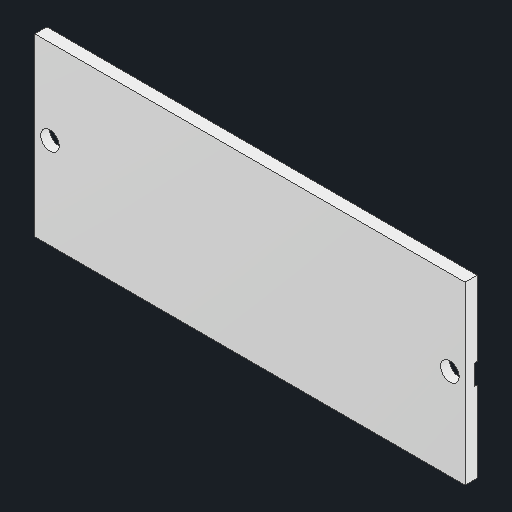
# Autodesk Inventor part: back
Saved by Autodesk Inventor 2023 (Build 270158000, 158)
## iProperties
Created: 2024-05-26
Part Number: back
Material: ABS Plastic
Document SubType Name: Modeling
Designer: szymo
Density: 1.06 g/cm^3
Appearance: Smooth - White
Mass: 4.30907 g
Surface Area: 45.139 cm^2
Volume: 4.06516 cm^3
TOTAL MASS: 0.0
Author: szymo
Autodesk Inventor part; units mm, degrees
ref_plane "YZ Plane" through (0, 0, 0) normal (1, 0, 0) x (0, 1, 0)
ref_plane "XZ Plane" through (0, 0, 0) normal (0, 1, 0) x (-1, 0, 0)
ref_plane "XY Plane" through (0, 0, 0) normal (0, 0, 1) x (1, 0, 0)
sketch "Sketch3" plane through (0, 0, 0) normal (0, 0, 1) x (1, 0, 0)
  line L0 (2.676, 4.0583) -> (2.676, 33.0583) projected
  line L1 (2.676, 4.0583) -> (-2.324, 4.0583) projected
  line L2 (-2.324, 4.0583) -> (-2.324, 33.0583) projected
  line L3 (2.676, 33.0583) -> (-2.324, 33.0583) projected
  line L4 (-68.324, 4.0583) -> (-68.324, 29.5583) projected
  line L5 (-68.324, 33.0583) -> (-63.324, 33.0583) projected
  line L6 (-63.324, 4.0583) -> (-63.324, 33.0583) projected
  line L7 (-68.324, 4.0583) -> (-63.324, 4.0583) projected
  line L8 (2.676, 33.0583) -> (-68.324, 33.0583)
  line L9 (-68.324, 33.0583) -> (-68.324, 4.0583)
  line L10 (-68.324, 4.0583) -> (2.676, 4.0583)
  line L11 (2.676, 4.0583) -> (2.676, 33.0583)
  circle A0 centre (0.176, 19.0583) radius 1.75 projected
  line L12 (-68.324, 29.5583) -> (-68.324, 33.0583) projected
  circle A1 centre (-65.824, 19.0583) radius 1.75 projected
  point P0 (0, 0)
  constraints: 8 end point, 2 parallel, 1 horizontal, 1 perpendicular
extrude "Extrusion2" add sketch "Sketch3" against normal blind 2 contours L1 L2 L3 L0 | L10 L6 L8 L2 | L7 L4 L9 L5 L6 | A0 | A1
sketch "Sketch4" plane through (0, 0, -2) normal (0, 0, -1) x (-1, 0, 0)
  circle A0 centre (-0.176, 19.0583) radius 1.75 projected
  circle A1 centre (65.824, 19.0583) radius 1.75 projected
  point P0 (0, 0)
  constraints: 2 coincident
hole "Hole2" at (0.176, 19.0583, -2) at (-65.824, 19.0583, -2) direction (0, 0, 1) diameter 3.1 end through all counterbore diameter 6 counterbore depth 0.5 clearance for "Countersunk Flat Head Screw ISO 2009/7046" size "M2.5" standard "ISO"
body "Solid2"
